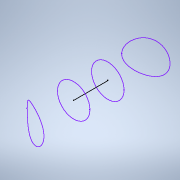
# Autodesk Inventor part: HandleRod1
Saved by Autodesk Inventor 2021 (Build 250183000, 183)
## iProperties
Created: 2021-06-03
Part Number: HandleRod1
Material: Generic
Document SubType Name: Modeling
Designer: teh18
Density: 1 g/cm^3
Appearance: Default
Author: teh18
Autodesk Inventor part; units mm, degrees
ref_plane "YZ Plane" through (0, 0, 0) normal (1, 0, 0) x (0, 1, 0)
ref_plane "XZ Plane" through (0, 0, 0) normal (0, 1, 0) x (-1, 0, 0)
ref_plane "XY Plane" through (0, 0, 0) normal (0, 0, 1) x (1, 0, 0)
ref_plane "Work Plane4" through (66.1421, 0, 10) normal (0, 0, -1) x (-1, 0, 0)
ref_plane "Work Plane2" through (66.1421, 0, 20) normal (0, 0, -1) x (-1, 0, 0)
ref_plane "Work Plane3" through (0, 0, 0) normal (0, 0, 1) x (1, 0, 0)
sketch "Sketch3" plane through (66.1421, 0, 10) normal (0, 0, -1) x (-1, 0, 0)
  circle A0 centre (51.9367, 20) radius 9.525 projected
  point P0 (66.1421, 0)
extrude "Extrusion1" add sketch "Sketch3" along normal mid plane 80
sketch "Sketch4" plane through (14.2054, 20, 50) normal (0, 0, 1) x (1, 0, 0)
  circle A0 centre (0, 0) radius 9.525 projected
  point P0 (-14.2054, -20)
ref_plane "Work Plane5" through (29.321, 40, 10) normal (0, 1, 0) x (-1, 0, 0)
sketch "Sketch5" plane through (29.321, 40, 10) normal (0, 1, 0) x (-1, 0, 0)
  line L0 (-36.821, 10) -> (29.321, 10) projected
  line L1 (29.321, 10) -> (29.321, -10) projected
  line L2 (29.321, -10) -> (-36.821, -10) projected
  arc A0 (-36.821, -10) -> (34.3068, -13.5) centre (-0.679, 0) ccw projected
  line L3 (34.3068, -13.5) -> (39.3068, -13.5) projected
  line L4 (39.3068, -13.5) -> (43.0149, 0) projected
  line L5 (43.0149, 0) -> (39.3068, 13.5) projected
  line L6 (39.3068, 13.5) -> (34.3068, 13.5) projected
  arc A1 (34.3068, 13.5) -> (-36.821, 10) centre (-0.679, 0) ccw projected
  line L7 (5.5907, -10) -> (24.6407, -10) projected
  line L8 (5.5907, -10) -> (24.6407, -10) projected
  line L9 (24.6407, 10) -> (5.5907, 10) projected
  arc A2 (2.1162, -37.3957) -> (28.5539, -23.4881) centre (-0.679, 0) ccw
  arc A3 (28.5539, 23.4881) -> (2.1162, 37.3957) centre (-0.679, 0) ccw
  line L10 (28.5539, -66.6217) -> (28.5539, -23.4881)
  line L11 (28.5539, 23.4881) -> (28.5539, 69.2229)
  line L12 (2.1162, -66.6217) -> (2.1162, -37.3957)
  line L13 (2.1162, 37.3957) -> (2.1162, 69.2229)
  line L14 (28.5539, -66.6217) -> (2.1162, -66.6217)
  line L15 (28.5539, 69.2229) -> (2.1162, 69.2229)
  point P0 (28.5539, -23.4881)
  point P1 (2.1162, -37.3957)
  point P2 (2.1162, 37.3957)
  constraints: 14 end point, 4 point on circle, 4 vertical, 2 centre point, 1 coincident, 1 horizontal, 1 parallel
extrude "Extrusion2" cut sketch "Sketch5" against normal blind 30 contours L13 L15 L11 A1 | A0 L10 L14 L12
body "Solid1"
